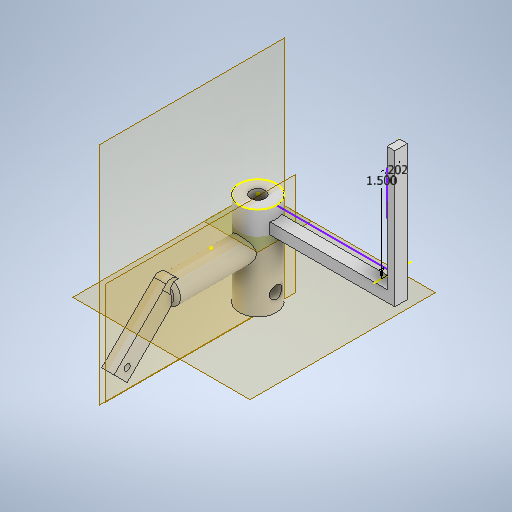
# Autodesk Inventor part: NEWYORKWHEELS
Saved by Autodesk Inventor 2025 (Build 290162010, 162A)
## iProperties
Created: 2024-07-31
Part Number: NEWYORKWHEELS
Material: Generic
Document SubType Name: Modeling
Designer: darkb
Density: 1 g/cm^3
Appearance: Default
Author: darkb
Autodesk Inventor part; units mm, degrees
ref_plane "XY Plane" through (0, 0, 0) normal (0, 0, 1) x (1, 0, 0)
sketch "Sketch1" plane through (0, 0, 0) normal (0, 1, 0) x (-1, 0, 0)
  circle A0 centre (0, 0) radius 9.2486
  circle A1 centre (0, 0) radius 2.9781
  dimension "d0" = 5.9563
  constraints: 2 centre point, 2 coincident
  measures "d0" diameter of A1
ref_plane "Work Plane2" through (0, 0, 0) normal (0, -1, 0) x (1, 0, 0)
sketch "Sketch2" plane through (0, 0, 0) normal (0, -1, 0) x (1, 0, 0)
  circle A0 centre (0, 0) radius 3.81
  dimension "d4" = 7.62
  constraints: 1 centre point, 1 coincident
  measures "d4" diameter of A0
extrude "Extrusion2" add sketch "Sketch2" along normal blind 19.05
sketch "Sketch3" plane through (0, -19.05, 0) normal (0, -1, 0) x (1, 0, 0)
  point P0 (0, 0)
sketch "Sketch5" plane through (0, 0, 0) normal (0, 0, 1) x (1, 0, 0)
  point P0 (0, 0)
sketch "Sketch6" plane through (0, 0, 0) normal (0, 0, 1) x (1, 0, 0)
  circle A0 centre (0, -7.8887) radius 2.54
  point P0 (0, 0)
  dimension "d12" = 5.08
  constraints: 1 centre point
  measures "d12" diameter of A0
extrude "Extrusion4" add sketch "Sketch6" along normal blind 19.05
chamfer "Chamfer1" distance 0.6731 angle 45 1 edges at (-2.54, -7.8887, 19.05)
sketch "Sketch7" plane through (0, -7.8887, 19.05) normal (0, 0, 1) x (1, 0, 0)
  point P0 (0, 7.8887)
sketch "Sketch8" plane through (0, -7.8887, 19.05) normal (0, 0, 1) x (1, 0, 0)
  point P0 (0, 7.8887)
sketch "Sketch9" plane through (0, 0, 0) normal (1, 0, 0) x (0, 1, 0)
  line L0 (-10.4287, 3.81) -> (-10.4287, 18.3769) projected
  line L1 (-9.7556, 19.05) -> (-6.0218, 19.05) projected
  line L2 (-10.4287, 18.3769) -> (-9.7556, 19.05)
  line L3 (-9.7556, 19.05) -> (-18.7359, 28.0303)
  line L4 (-18.7359, 28.0303) -> (-16.0418, 30.7243)
  line L5 (-16.0418, 30.7243) -> (-6.0218, 20.7044)
  line L6 (-6.0218, 20.7044) -> (-8.7159, 18.0103)
  line L7 (-8.7159, 18.0103) -> (-10.4287, 19.7231)
  point P0 (0, 0)
  point P1 (-7.6762, 19.05)
  dimension "d18" = 12.7
  dimension "d19" = 3.81
  constraints: 12 end point, 3 perpendicular, 2 point on line
  measures "d18" distance of L1.start L3.end
  measures "d19" distance of L3.end L4.end
extrude "Extrusion5" add sketch "Sketch9" along normal mid plane 2.54 contours L3 L4 L5 L6 L1
sketch "Sketch10" plane through (-1.27, -16.0418, 30.7243) normal (0, 0.7071068, 0.7071068) x (1, 0, 0)
  line L0 (0, 14.1704) -> (2.54, 14.1704) projected
  line L1 (0, 14.1704) -> (2.463, 14.1704)
  line L2 (2.463, 14.1704) -> (2.463, 16.7542)
  line L3 (2.463, 16.7542) -> (0, 16.7542)
  line L4 (0, 16.7542) -> (0, 14.1704)
  point P0 (1.27, 33.0687)
  dimension "d22" = 2.5838
  constraints: 8 end point, 2 parallel, 1 horizontal, 1 perpendicular
  measures "d22" distance of L3.end L0.start
extrude "Extrusion6" add sketch "Sketch10" against normal blind 2.54
scale "Scale1" factors (2, 2, 2) then translate (0, 9.525, 0) bodies 1
fillet "Fillet2" radius 3.175 1 edges at (-0.077, 1.1354, 37.7546)
sketch "Sketch15" plane through (0, 0, 0) normal (1, 0, 0) x (0, 1, 0)
  point P0 (0, 0)
sketch "Sketch16" plane through (0, -28.575, 0) normal (0, -1, 0) x (1, 0, 0)
  circle A0 centre (0, 0) radius 2.54
  dimension "d38" = 5.08
  constraints: 1 centre point, 1 coincident
  measures "d38" diameter of A0
extrude "Extrusion10" cut sketch "Sketch16" along normal mid plane 254
ref_plane "Work Plane3" through (2.54, 0, 0) normal (1, 0, 0) x (0, 1, 0)
sketch "Sketch17" plane through (0, 0, 0) normal (1, 0, 0) x (0, 1, 0)
  circle A0 centre (-21.3519, 0) radius 2.54
  point P0 (0, 0)
  dimension "d42" = 5.08
  constraints: 1 centre point
  measures "d42" diameter of A0
extrude "Extrusion11" cut sketch "Sketch17" along normal blind 254
sketch "Sketch18" plane through (2.54, -8.9892, 38.1) normal (1, 0, 0) x (0, 0, -1)
  circle A0 centre (-17.9605, -13.5694) radius 1.27
  point P0 (38.1, 8.9892)
  dimension "d45" = 2.54
  constraints: 1 centre point
  measures "d45" diameter of A0
extrude "Extrusion12" cut sketch "Sketch18" along normal mid plane 254
sketch "Sketch20" plane through (2.54, 0, 0) normal (1, 0, 0) x (0, 1, 0)
  line L0 (4.5821, 2.3169) -> (0, 2.3169)
  line L1 (0, 2.3169) -> (0, -2.8151)
  line L2 (0, -2.8151) -> (4.5821, -2.8151)
  line L3 (4.5821, -2.8151) -> (4.5821, 2.3169)
  point P0 (0, 0)
  constraints: 8 end point, 2 parallel, 1 horizontal, 1 perpendicular
extrude "Extrusion13" add sketch "Sketch20" along normal blind 55.88
sketch "Sketch21" plane through (7.0809, 4.5821, -2.8151) normal (0, 1, 0) x (1, 0, 0)
  point P0 (-7.0809, -2.8151)
sketch "Sketch22" plane through (7.0809, 4.5821, -2.8151) normal (0, 1, 0) x (1, 0, 0)
  line L0 (0, 0) -> (51.3391, 0) projected
  line L1 (0.1783, -5.1319) -> (51.3391, -5.1319) projected
  line L2 (48.2036, 0) -> (51.3391, 0)
  line L3 (51.3391, 0) -> (51.3391, -5.1319)
  line L4 (51.3391, -5.1319) -> (48.2036, -5.1319)
  line L5 (48.2036, -5.1319) -> (48.2036, 0)
  point P0 (-7.0809, -2.8151)
  constraints: 8 end point, 2 parallel, 1 horizontal, 1 perpendicular, 1 point on line
extrude "Extrusion14" add sketch "Sketch22" along normal blind 50.8
sketch "Sketch23" plane through (55.2846, 4.5821, -2.8151) normal (-1, 0, 0) x (0, 0, 1)
  line L0 (0, 0) -> (0, 50.8) projected
  line L1 (5.1308, 43.0429) -> (0, 43.0429)
  line L2 (0, 43.0429) -> (0, 19.9713)
  line L3 (0, 25.4607) -> (5.1308, 25.4607)
  line L4 (5.1308, 25.4607) -> (5.1308, 43.0429)
  line L5 (-4.8049, 4.9429) -> (10.4351, 4.9429) projected
  point P0 (2.8151, -4.5821)
  point P1 (0, 43.0429)
  point P2 (0, 25.4607)
  dimension "d54" = 38.1
  dimension "d55" = 5.1308
  constraints: 8 end point, 2 parallel, 1 horizontal, 1 perpendicular
  measures "d54" distance between parallel lines of L1 L5
  measures "d55" distance of L1.start L1.end
sketch "Sketch24" plane through (0, 9.525, 0) normal (0, 1, 0) x (1, 0, 0)
  circle A0 centre (0, 0) radius 7.62 projected
  line L0 (7.62, 0) -> (55.2846, 0)
  line L1 (55.2846, 2.8151) -> (55.2846, -2.3169) projected
  constraints: 2 end point, 1 horizontal, 1 horizontal alignment, 1 point on line, 1 other
sketch "Sketch25" plane through (58.42, 0, -2.8151) normal (0, 0, -1) x (-1, 0, 0)
  line L0 (3.1354, 4.5821) -> (3.1354, 55.3821) projected
  line L1 (3.1354, 19.685) -> (3.1354, 24.5529)
  line L2 (3.1354, 4.5821) -> (3.1354, 55.3821) projected
  point P0 (58.42, 0)
  point P1 (3.1354, 30.0428)
  constraints: 2 end point, 1 point on line
sketch "Sketch28" plane through (55.2846, 55.3821, -2.8151) normal (-1, 0, 0) x (0, 0, 1)
  point P0 (2.8151, -55.3821)
extrude "Extrusion19" cut sketch "Sketch1" along normal mid plane 254 contours A1
body "Solid1"
